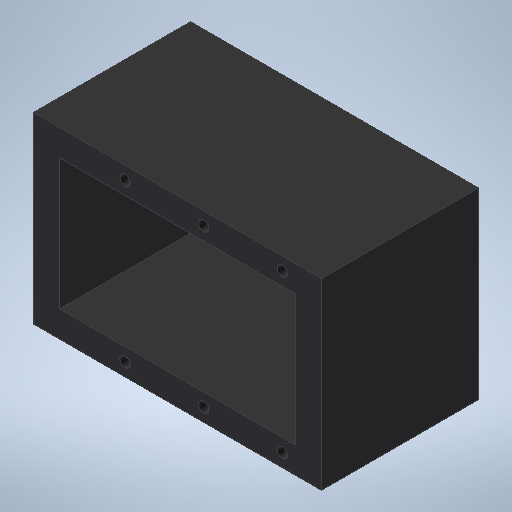
# Autodesk Inventor part: ESP box
Saved by Autodesk Inventor 2025 (Build 290162000, 162)
## iProperties
Created: 2025-11-29
Part Number: ESP box
Material: Generic
Document SubType Name: Modeling
Designer: ruven
Density: 1 g/cm^3
Appearance: Default
Author: ruven
Autodesk Inventor part; units mm, degrees
ref_plane "YZ Plane" through (0, 0, 0) normal (1, 0, 0) x (0, 1, 0)
ref_plane "XZ Plane" through (0, 0, 0) normal (0, 1, 0) x (-1, 0, 0)
ref_plane "XY Plane" through (0, 0, 0) normal (0, 0, 1) x (1, 0, 0)
sketch "Sketch1" plane through (0, 0, 0) normal (0, 1, 0) x (-1, 0, 0)
  line L0 (55, 25) -> (55, -25)
  line L1 (-55, 25) -> (55, -25) construction
  line L2 (55, 25) -> (-55, -25) construction
  line L3 (-45, 35) -> (65, 35)
  line L4 (65, 35) -> (65, -35)
  line L5 (65, -35) -> (-45, -35)
  line L6 (-65, 35) -> (65, -35) construction
  line L7 (65, 35) -> (-65, -35) construction
  circle A0 centre (30, 30) radius 2
  circle A1 centre (0, 30) radius 2
  circle A2 centre (-30, 30) radius 2
  line L8 (55, 0) -> (-55, 0) construction
  circle A3 centre (30, -30) radius 2
  circle A4 centre (0, -30) radius 2
  circle A5 centre (-30, -30) radius 2
  line L9 (-35, 25) -> (-35, -25)
  line L10 (-45, -35) -> (-45, 35)
  line L11 (-35, 25) -> (55, 25)
  line L12 (55, -25) -> (-35, -25)
  point P0 (0, 0)
  point P1 (0, 25)
  point P2 (0, 35)
  dimension "d4" = 4
  dimension "d5" = 4
  dimension "d6" = 4
  dimension "d7" = 30
  dimension "d8" = 30
  dimension "d9" = 0
  dimension "d16" = 60
  dimension "d18" = 70
  dimension "d19" = 10
  dimension "d20" = 5
  constraints: 26 end point, 6 centre point, 5 midpoint, 4 perpendicular, 3 symmetric about line, 2 horizontal, 2 parallel, 2 point on line, 3 other
  measures "d4" diameter of A0
  measures "d5" diameter of A1
  measures "d6" diameter of A2
  measures "d7" distance of A0.centre A1.centre
  measures "d8" distance between centres of A2 A1
  measures "d9" horizontal distance of point (0, 25) A1.centre
  measures "d16" distance of A3.centre A0.centre
  measures "d18" distance from line of L5 point (0, 35)
  measures "d19" distance between parallel lines of L10 L9
  measures "d20" distance from line of A2.centre L9
extrude "Extrusion1" add sketch "Sketch1" along normal blind 60
body "Solid1"
